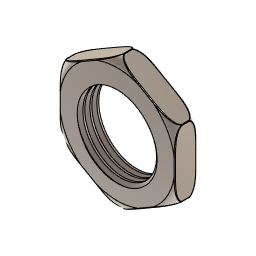
Inductive_Proximity_Nut_Fastener (Autodesk Fusion 360 design; units mm, degrees)
Autodesk Fusion 360 part; units mm, degrees
note: some values were not read from the file. Set by a fixed rule: which sketch regions a step uses.
sketch "Sketch1" plane through (0, 0, 0) normal (0, 1, 0) x (1, 0, 0)
  circle A0 centre (0, 0) radius 9.55
  circle A1 centre (0, 0) radius 5.5
  dimension "d1" = 19.1
  dimension "d2" = 11
  constraint coincident A0.centre A1.centre
  constraint concentric A0 A1
  measures "d1" diameter of A0
  measures "d2" diameter of A1
extrude "Extrude1" add sketch "Sketch1" along normal mid plane 3.1
fillet "Fillet1" radius 1.3 2 edges at (-8.9037, -1.55, -3.4534) (-8.9037, 1.55, 3.4534)
sketch "Sketch2" plane through (0, -1.55, 0) normal (0, -1, 0) x (1, 0, 0)
  circle A0 centre (0, 0) radius 5.5
  circle A1 centre (0, 0) radius 8.25
  line L0 (-8.25, -4.7631) -> (0, -9.5263)
  line L1 (0, -9.5263) -> (8.25, -4.7631)
  line L2 (8.25, -4.7631) -> (8.25, 4.7631)
  line L3 (8.25, 4.7631) -> (0, 9.5263)
  line L4 (0, 9.5263) -> (-8.25, 4.7631)
  line L5 (-8.25, 4.7631) -> (-8.25, -4.7631)
  dimension "d7" = 8.25
  constraint coincident A0.centre A1.centre
  measures "d7" distance of A0.centre L5
extrude "Extrude2" cut sketch "Sketch2" against normal blind 4 keep common part
fillet "Fillet2" radius 0.1 30 edges at (-1.9044, 1.4912, 8.4268) (-6.3456, 1.4912, 5.8626) (-6.3456, -1.4912, 5.8626) (-1.9044, -1.4912, 8.4268) (-8.25, 1.4918, 2.5665) (-8.25, 1.4918, -2.5665) (-8.25, -1.4918, -2.5665) (-8.25, -1.4918, 2.5665) (-8.25, 0, 4.7631) (-8.25, 0, -4.7631) (-6.3456, 1.4912, -5.8626) (-1.9044, 1.4912, -8.4268) (-1.9044, -1.4912, -8.4268) (-6.3456, -1.4912, -5.8626) (0, 0, -9.5263) (6.3477, -1.4918, -5.8615) (1.9023, -1.4918, -8.428) (1.9023, 1.4918, -8.428) (6.3477, 1.4918, -5.8615) (8.25, -1.4918, 2.5665) (8.25, -1.4918, -2.5665) (8.25, 1.4918, -2.5665) (8.25, 1.4918, 2.5665) (8.25, 0, -4.7631) (8.25, 0, 4.7631) (1.9023, -1.4918, 8.428) (6.3477, -1.4918, 5.8615) (6.3477, 1.4918, 5.8615) (1.9023, 1.4918, 8.428) (0, 0, 9.5263)
thread "Thread1" "ISO Metric profile 12.0 M12x1 6H" major diameter 12.152 minor diameter 11.035 pitch 1 angle 60 modelled right hand crest width 0.2719 on face at (5.4932, 0.5167, 0.2742) crest through (5.5175, -1.3, 0)
equation "d7 = ( 16.5 / 2 ) * 1 mm"
